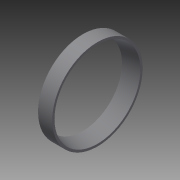
# Autodesk Inventor part: 32912_or
Saved by Autodesk Inventor 2014 SP2 (Build 180246200, 246)
## iProperties
Created: 2018-11-12
Part Number: 32912_or
Material: Generic
Catalog Web Link: www.cadenas.de
Description: BT1_001_101_or-Tapered roller bearings, single row
Vendor: SKF
Document SubType Name: Modeling
Designer: psadmin
Manufacturer: SKF
Mass: 13.3548 g
Surface Area: 90.2963 cm^2
Volume: 13.3548 cm^3
Density: 1 g/cm^3
Appearance: PSOLRGB-175-175-175
Category: PARTsolutions
Company: SKF
Title: 32912_or
Author: Cadenas PARTsolutions
Comments: Tapered roller bearings, single row
PSOL_IDENT_0: {$CADENAS_DATA\23d-libs\skf\bearings_units_and_housings\roller_bearings\tapered_roller_bearings\tape
PSOL_IDENT_1: red_roller_bearings_single_row\parts\bt1_001_101_or.prj},166 {VTYP=3D},{NB=32912_or},{LINA=32912_or}
PSOL_IDENT_2: ,{NN=BT1_001_101_or},{DATE=14.08.2018 07:35:10},{GEOMDATE=29.05.2018 10:14:05},{VERSION=},{LINEID=21
PSOL_IDENT_3: 40},{WBVAR=},{WBNUMERIC=}  {NB=32912_or},{LINA=32912_or},{KT=DUMMY},{DESIGNATION=32912},{DD=60.000},
PSOL_IDENT_4: {D=85.000},{T=17.000},{DD1=73.8000},{D1=MIN},{B=17.000},{C=14.000},{C1=MIN},{R12=1.0},{R34=1.0},{AA=
PSOL_IDENT_5: 15.45165},{PITCH=72.347},{DW=5.200},{LW=12.200},{RANGLE=1.600},{ALPHA=12.450},{DDAMAX=67},{DDAMIN=68
PSOL_IDENT_6: .0},{DAMIN=78},{DAMAX=78.0},{DBMIN=81},{CA=3},{CB=3.0},{RA=1.0},{RB=1.0},{LOAD1=53.200},{LOAD2=75.00
PSOL_IDENT_7: 0},{LOAD3=7.800},{SPEED1=6000},{SPEED2=7000},{EE=0.33},{Y=1.80},{Y0=1.0},{Y1=0},{X1=1},{X2=0.4},{X0=
PSOL_IDENT_8: 0.5},{Z=34},{II=1},{R1=0.00000231},{R2=10.9},{S1=0.009},{S2=2},{KZ=6},{KL=0.7},{BF=2},{MASS=0.302},{
PSOL_IDENT_9: PIM=PIM_BT1_001},{DESIGN=trb1},{HELP=0.000}
NN: BT1_001_101_or
NT: Tapered roller bearings, single row
NB: 32912_or
NBSYN: $DESIGNATION._or
LINA: 32912_or
DESIGNATION: 32912
DD: 60
D: 85
T: 17
DD1: 73.8
D1: 0
B: 17
C: 14
C1: 0
R12: 1
R34: 1
AA: 15.45165
PITCH: 72.347
DW: 5.2
LW: 12.2
RANGLE: 1.6
ALPHA: 12.45
DDAMAX: 67
DDAMIN: 68
DAMIN: 78
DAMAX: 78
DBMIN: 81
CA: 3
CB: 3
RA: 1
RB: 1
LOAD1: 53.2
LOAD2: 75
LOAD3: 7.8
SPEED1: 6000
SPEED2: 7000
EE: 0.33
Y: 1.8
Y0: 1
Y1: 0
X1: 1
X2: 0.4
X0: 0.5
Z: 34
II: 1
R1: 0.00000231
R2: 10.9
S1: 0.009
S2: 2
KZ: 6
KL: 0.7
BF: 2
MASS: 0.302
PIM: PIM_BT1_001
SUPPLIER: SKF
ARTICLENO: 32912_or
BOMINFO: 32912_or
CREATOR: CADENAS GmbH
Autodesk Inventor part; units mm, degrees
sketch "Sketch_1" plane through (0, 0, 0) normal (0, 0, 1) x (1, 0, 0)
  line L0 (14, 0) -> (1, 0)
  line L1 (0, 41.5) -> (0, 37.0753)
  line L2 (0, 37.0753) -> (14, 40.3945)
  line L3 (14, 40.3945) -> (14, 42.5)
  line L4 (14, 42.5) -> (1, 42.5)
  arc A0 (1, 42.5) -> (0, 41.5) centre (1, 41.5) ccw
  constraints: 10 end point, 2 point on circle, 1 centre point
revolve "Revolution1" add sketch "Sketch_1" angle 360 about axis through (14, 0, 0) along (1, 0, 0)
ref_plane "outer_ring_XY" through (0, 0, 0) normal (0, 0, 1) x (1, 0, 0)
ref_plane "outer_ring_YZ" through (0, 0, 0) normal (1, 0, 0) x (0, 1, 0)
ref_plane "outer_ring_ZX" through (0, 0, 0) normal (0, 1, 0) x (0, 0, 1)
body "Solid1"
